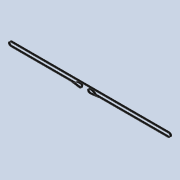
# Autodesk Inventor part: 0005-10-1016 curea Y
Saved by Autodesk Inventor 2020 (Build 240168000, 168)
## iProperties
Created: 2020-12-19
Part Number: 0005-10-1016 curea Y
Material: Generic
Document SubType Name: Modeling
Designer: Iulian Bors
Density: 1 g/cm^3
Appearance: Default(1)
Mass: 6.55704 g
Surface Area: 152.998 cm^2
Volume: 6.55704 cm^3
Author: Iulian Bors
Subject: 10-1016
Autodesk Inventor part; units mm, degrees
ref_plane "YZ Plane" through (0, 0, 0) normal (1, 0, 0) x (0, 1, 0)
ref_plane "XZ Plane" through (0, 0, 0) normal (0, 1, 0) x (-1, 0, 0)
ref_plane "XY Plane" through (0, 0, 0) normal (0, 0, 1) x (1, 0, 0)
sketch "Sketch1" plane through (0, 0, 0) normal (0, 0, 1) x (1, 0, 0)
  line L0 (-260.6545, 0) -> (265.3455, 0) construction
  line L1 (-260.6545, -6) -> (265.3455, -6)
  line L2 (265.3455, 6) -> (-260.6545, 6)
  arc A0 (-260.6545, 6) -> (-260.6545, -6) centre (-260.6545, 0) ccw
  arc A1 (265.3455, -6) -> (265.3455, 6) centre (265.3455, 0) ccw
  line L3 (-260.6545, 7) -> (265.3455, 7)
  arc A2 (265.3455, -7) -> (265.3455, 7) centre (265.3455, 0) ccw
  line L4 (265.3455, -7) -> (-260.6545, -7)
  arc A3 (-260.6545, 7) -> (-260.6545, -7) centre (-260.6545, 0) ccw
  point P0 (0, 0)
  point P1 (2.3455, 0)
  dimension "d0" = 526
  dimension "d1" = 12
  dimension "d2" = 1
  constraints: 12 end point, 8 point on circle, 4 centre point, 4 tangent, 2 parallel, 1 horizontal, 1 midpoint, 3 other
  measures "d0" distance of L0.start L0.end
  measures "d1" distance between parallel lines of L1 L2
  measures "d2" distance between parallel lines of L2 L3
extrude "Extrusion1" add sketch "Sketch1" along normal mid plane 6
sketch "Sketch7" plane through (-260.6545, -7, 3) normal (0, -1, 0) x (1, 0, 0)
  line L0 (221.6418, 58.3771) -> (221.6418, -71.6229) projected
  line L1 (409.1418, -121.6229) -> (409.1418, 108.3771) projected
  line L2 (211.6418, 0) -> (281.6418, 0)
  line L3 (281.6418, 0) -> (281.6418, -6)
  line L4 (281.6418, -6) -> (211.6418, -6)
  line L5 (211.6418, -6) -> (211.6418, 0)
  line L6 (0, 0) -> (526, 0) projected
  line L7 (526, -6) -> (0, -6) projected
  line L8 (271.6418, -71.6229) -> (271.6418, 58.3771) projected
  point P0 (260.6545, -3)
  dimension "d11" = 10
  dimension "d17" = 10
  constraints: 8 end point, 2 collinear, 2 parallel, 1 horizontal, 1 perpendicular
  measures "d11" distance between parallel lines of L0 L5
  measures "d17" distance between parallel lines of L8 L3
extrude "Extrusion3" cut sketch "Sketch7" against normal blind 10 contours L2 L8 L4 L0 | L0 L4 L5 L2 | L2 L3 L4 L8
sketch "Sketch8" plane through (0, 0, 0) normal (0, 0, 1) x (1, 0, 0)
  line L0 (-39.0127, -8.8612) -> (-39.0127, -0.8612) projected
  line L1 (-29.0127, -8.8612) -> (-29.0127, -0.8612) projected
  line L2 (-49.0127, -6) -> (-49.0127, -7) projected
  line L3 (-49.0127, -7) -> (-49.0127, -6) projected
  line L4 (-49.0127, -6.5) -> (-46.6485, -5.141) construction
  line L5 (-46.6485, -5.141) -> (-43.2177, -1.1048) construction
  line L6 (-43.2177, -1.1048) -> (-37.7352, 1.2833) construction
  line L7 (-37.7352, 1.2833) -> (-27.9473, 1.5524) construction
  line L8 (-27.9473, 1.5524) -> (-24.2474, 0.6779) construction
  line L9 (-24.2474, 0.6779) -> (-24.2474, -3.0893) construction
  line L10 (-24.2474, -3.0893) -> (-24.5501, -9.0427) construction
  line L11 (-24.5501, -9.0427) -> (-26.9382, -11.4981) construction
  line L12 (-26.9382, -11.4981) -> (-30.5372, -11.2963) construction
  line L13 (-30.5372, -11.2963) -> (-37.8697, -10.3545) construction
  line L14 (-37.8697, -10.3545) -> (-48.6666, -8.1346) construction
  line L15 (-48.6666, -8.1346) -> (-55.7637, -7.8655) construction
  spline S0 degree 4 poles (-49.0127, -6.5) (-46.6485, -5.141) (-43.2177, -1.1048) (-37.7352, 1.2833) (-27.9473, 1.5524) (-24.2474, 0.6779) (-24.2474, -3.0893) (-24.5501, -9.0427) (-26.9382, -11.4981) (-30.5372, -11.2963) (-37.8697, -10.3545) (-48.6666, -8.1346) (-55.7637, -7.8655) knots 1 1 1 1 1 2 3 4 5 6 7 8 9 10 10 10 10 10
  point P0 (0, 0)
  constraints: 1 midpoint, 1 parallel, 3 other
sketch "Sketch9" plane through (-49.0127, -7, 3) normal (1, 0, 0) x (0, 0, -1)
  line L0 (0, 1) -> (6, 1) projected
  line L1 (0, 0) -> (0, 1) projected
  line L2 (6, 0) -> (0, 0) projected
  line L3 (6, 1) -> (6, 0) projected
  point P0 (3, 7)
sweep "Sweep3" add profiles "Sketch9" path "Sketch8" separate body path curves S0
sketch "Sketch10" plane through (0, 0, 0) normal (0, 0, 1) x (1, 0, 0)
  line L0 (10.9873, -8.8612) -> (10.9873, -0.8612) projected
  line L1 (0.9873, -8.8612) -> (0.9873, -0.8612) projected
  line L2 (20.9873, -7) -> (20.9873, -6) projected
  line L3 (20.9873, -6) -> (20.9873, -7) projected
  line L4 (20.9873, -6.5) -> (14.1955, 0.6024) construction
  line L5 (14.1955, 0.6024) -> (7.3246, 1.5273) construction
  line L6 (7.3246, 1.5273) -> (-4.1709, 0.9988) construction
  line L7 (-4.1709, 0.9988) -> (-3.5102, -3.6259) construction
  line L8 (-3.5102, -3.6259) -> (-2.1228, -10.8931) construction
  line L9 (-2.1228, -10.8931) -> (5.3427, -10.8931) construction
  line L10 (5.3427, -10.8931) -> (15.5829, -9.9682) construction
  line L11 (15.5829, -9.9682) -> (23.0484, -8.8612) construction
  line L12 (23.0484, -8.8612) -> (30.3157, -7.6559) construction
  line L13 (30.3157, -7.6559) -> (32.7601, -7.6559) construction
  spline S0 degree 4 poles (20.9873, -6.5) (14.1955, 0.6024) (7.3246, 1.5273) (-4.1709, 0.9988) (-3.5102, -3.6259) (-2.1228, -10.8931) (5.3427, -10.8931) (15.5829, -9.9682) (23.0484, -8.8612) (30.3157, -7.6559) (32.7601, -7.6559) knots 1 1 1 1 1 2 3 4 5 6 7 8 8 8 8 8
  point P0 (0, 0)
  constraints: 2 perpendicular, 1 midpoint, 3 other
sketch "Sketch11" plane through (20.9873, -7, -3) normal (-1, 0, 0) x (0, 0, 1)
  line L0 (0, 1) -> (6, 1) projected
  line L1 (0, 0) -> (0, 1) projected
  line L2 (6, 0) -> (0, 0) projected
  line L3 (6, 1) -> (6, 0) projected
  point P0 (3, 7)
sweep "Sweep4" add profiles "Sketch11" path "Sketch10" separate body path curves S0
equation "\"d17\" = d11"
body "Solid1"
body "Solid4"
body "Solid5"
